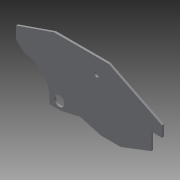
# Autodesk Inventor part: ShooterMountLeft_NERDS
Saved by Autodesk Inventor 2014 (Build 180170000, 170)
## iProperties
Created: 2016-01-30
Part Number: ShooterMountLeft_NERDS
Material: Generic
Document SubType Name: Modeling
Designer: bermudezr
Density: 1 g/cm^3
Appearance: Default
Author: bermudezr
Autodesk Inventor part; units mm, degrees
ref_plane "YZ Plane" through (0, 0, 0) normal (1, 0, 0) x (0, 1, 0)
ref_plane "XZ Plane" through (0, 0, 0) normal (0, 1, 0) x (-1, 0, 0)
ref_plane "XY Plane" through (0, 0, 0) normal (0, 0, 1) x (1, 0, 0)
sketch "Sketch1" plane through (0, 0, 0) normal (0, 0, 1) x (1, 0, 0)
  line L0 (-84.0821, 192.7052) -> (642.9929, 192.7052)
  line L1 (642.9929, 192.7052) -> (642.9929, -137.4948)
  line L2 (642.9929, -137.4948) -> (-84.0821, -137.4948)
  line L3 (-84.0821, -137.4948) -> (-84.0821, 192.7052)
  circle A0 centre (131.8179, -91.7748) radius 25.4
  circle A1 centre (318.0537, 116.5052) radius 12.7
  line L4 (642.9929, -137.4948) -> (592.1929, -137.4948)
  line L5 (592.1929, -137.4948) -> (592.1929, -73.9948)
  line L6 (592.1929, -73.9948) -> (642.9929, -73.9948)
  line L7 (642.9929, -73.9948) -> (642.9929, -137.4948)
  line L8 (642.9929, 192.7052) -> (592.6352, 192.7052)
  line L9 (642.9929, 2.2052) -> (642.9929, 192.7052)
  line L10 (-84.0821, 53.0052) -> (5.7204, 53.0052) construction
  line L11 (-84.0821, 65.7052) -> (68.3179, -137.4948)
  line L12 (595.3679, 192.7052) -> (595.3679, 2.2052)
  line L13 (595.3679, 2.2052) -> (642.9929, 2.2052)
  point P0 (0, 0)
  dimension "d0" = 727.075
  dimension "d2" = 50.8
  dimension "d3" = 25.4
  dimension "d4" = 215.9
  dimension "d5" = 279.4
  dimension "d14" = 152.4
  dimension "d15" = 203.2
  dimension "d16" = 330.2
  dimension "d17" = 63.5
  dimension "d19" = 50.8
  dimension "d20" = 139.7
  dimension "d21" = 45.72
  dimension "d22" = 254
  constraints: 28 end point, 5 parallel, 5 point on line, 4 horizontal, 3 perpendicular, 2 centre point
  measures "d0" distance of L1.end L2.end
  measures "d2" diameter of A0
  measures "d3" diameter of A1
  measures "d4" distance from line of L3 A0.centre
  measures "d5" distance of A1.centre A0.centre
  measures "d14" distance from line of L3 L11.end
  measures "d15" distance from line of L2 L11.start
  measures "d16" distance between parallel lines of L2 L0
  measures "d17" distance between parallel lines of L6 L2
  measures "d19" distance of L5.end L6.end
  measures "d20" distance between parallel lines of L13 L4
  measures "d21" distance from line of L2 A0.centre
  measures "d22" distance from line of L2 A1.centre
extrude "Extrusion1" add sketch "Sketch1" along normal blind 9.525 contours L0 L12 L13 L1 L6 L5 L2 L11 L3
sketch "Sketch3" plane through (0, 0, 9.525) normal (0, 0, 1) x (1, 0, 0)
  line L0 (595.3679, 2.2052) -> (595.3679, 192.7052) projected
  line L1 (595.3679, 192.7052) -> (-84.0821, 192.7052) projected
  line L2 (-84.0821, 192.7052) -> (-84.0821, 65.7052) projected
  line L3 (-84.0821, 127.1732) -> (106.4179, 192.7052)
  line L4 (595.3679, 2.2052) -> (684.2679, 2.2052)
  line L5 (684.2679, 2.2052) -> (684.2679, 40.3052)
  line L6 (684.2679, 40.3052) -> (595.3679, 40.3052)
  line L7 (595.3679, 40.3052) -> (595.3679, 2.2052)
  line L8 (684.2679, 40.3052) -> (379.4679, 192.7052)
  line L9 (595.3679, 40.3052) -> (595.3679, 84.7552)
  line L10 (595.3679, 84.7552) -> (595.3679, 192.7052)
  point P0 (0, 0)
  dimension "d32" = 190.5
  dimension "d33" = 65.532
  dimension "d38" = 88.9
  dimension "d39" = 38.1
  dimension "d40" = 215.9
  constraints: 16 end point, 5 point on line, 2 parallel, 1 collinear, 1 horizontal, 1 perpendicular
  measures "d32" distance from line of L2 L3.end
  measures "d33" distance from line of L1 L3.start
  measures "d38" distance of L6.end L5.end
  measures "d39" distance of L5.end L4.end
  measures "d40" distance of L0.end L8.end
extrude "Extrusion4" cut sketch "Sketch3" against normal blind 9.525 contours L3 L2 L1 | L8 L1 L0 | L0 L8 L6
sketch "Sketch4" plane through (0, 0, 9.525) normal (0, 0, 1) x (1, 0, 0)
  line L0 (595.3679, 2.2052) -> (595.3679, 84.7552) projected
  line L1 (595.3679, 84.7552) -> (379.4679, 192.7052) projected
  line L2 (595.3679, 84.7552) -> (684.2679, 40.3052)
  line L3 (684.2679, 40.3052) -> (595.3679, 40.3052)
  point P0 (0, 0)
  dimension "d43" = 88.9
  constraints: 4 end point, 1 collinear, 1 perpendicular, 1 point on line
  measures "d43" distance from line of L2.end L0
extrude "Extrusion5" add sketch "Sketch4" against normal blind 9.525
sketch "Sketch5" plane through (0, 0, 9.525) normal (0, 0, 1) x (1, 0, 0)
  line L0 (642.9929, 2.2052) -> (592.1929, 2.2052)
  line L1 (592.1929, 2.2052) -> (592.1929, -73.9948)
  line L2 (592.1929, -73.9948) -> (642.9929, -73.9948)
  line L3 (642.9929, -73.9948) -> (642.9929, 2.2052)
  point P0 (0, 0)
  constraints: 8 end point, 2 parallel, 1 horizontal, 1 perpendicular
extrude "Extrusion6" cut sketch "Sketch5" against normal blind 9.525
sketch "Sketch6" plane through (0, 0, 9.525) normal (0, 0, 1) x (1, 0, 0)
  line L0 (592.1929, -137.4948) -> (592.1929, 2.2052) projected
  line L1 (646.1679, 91.1052) -> (723.1394, 91.1052)
  line L2 (723.1394, 91.1052) -> (723.1394, -6.7385)
  line L3 (723.1394, -6.7385) -> (646.1679, -6.7385)
  line L4 (646.1679, -6.7385) -> (646.1679, 91.1052)
  line L5 (595.3679, 2.2052) -> (592.1929, 2.2052)
  line L6 (592.1929, 2.2052) -> (592.1929, 40.3052)
  line L7 (592.1929, 40.3052) -> (595.3679, 40.3052)
  line L8 (595.3679, 40.3052) -> (595.3679, 2.2052)
  point P0 (0, 0)
  dimension "d48" = 53.975
  constraints: 16 end point, 4 parallel, 2 horizontal, 2 perpendicular
  measures "d48" distance between parallel lines of L0 L4
extrude "Extrusion7" cut sketch "Sketch6" against normal blind 9.525
sketch "Sketch8" plane through (0, 0, 9.525) normal (0, 0, 1) x (1, 0, 0)
  line L0 (-84.0821, 65.7052) -> (68.3179, -137.4948) projected
  line L1 (68.3179, -137.4948) -> (592.1929, -137.4948) projected
  line L2 (592.1929, -137.4948) -> (592.1929, 40.3052) projected
  line L3 (592.1929, -96.6594) -> (439.7929, -137.4948)
  line L4 (341.7489, -137.4948) -> (170.3104, -117.1748)
  line L5 (170.3104, -117.1748) -> (53.0779, -117.1748)
  point P0 (0, 0)
  dimension "d51" = 152.4
  dimension "d52" = 165
  dimension "d53" = 98.044
  dimension "d54" = 20.32
  dimension "d60" = 173.24
  constraints: 6 end point, 4 point on line
  measures "d51" distance from line of L3.end L2
  measures "d52" angle of L1 L3
  measures "d53" distance of L3.end L4.start
  measures "d54" distance between parallel lines of L1 L5
  measures "d60" angle of L1 L4
extrude "Extrusion8" cut sketch "Sketch8" against normal blind 9.525
sketch "Sketch9" plane through (0, 0, 9.525) normal (0, 0, 1) x (1, 0, 0)
  line L0 (592.1929, -96.6594) -> (592.1929, 40.3052) projected
  line L1 (646.1679, 40.3052) -> (592.1929, 40.3052)
  line L2 (592.1929, 40.3052) -> (592.1929, 5.3802)
  line L3 (592.1929, 5.3802) -> (646.1679, 5.3802)
  line L4 (646.1679, 5.3802) -> (646.1679, 40.3052)
  point P0 (0, 0)
  dimension "d57" = 34.925
  constraints: 8 end point, 2 parallel, 1 horizontal, 1 perpendicular, 1 point on line
  measures "d57" distance of L2.end L1.end
extrude "Extrusion9" add sketch "Sketch9" against normal blind 9.525
sketch "Sketch10" plane through (0, 0, 9.525) normal (0, 0, 1) x (1, 0, 0)
  line L0 (-84.0821, 65.7052) -> (53.0779, -117.1748) projected
  line L1 (-84.0821, 127.1732) -> (-84.0821, 65.7052) projected
  line L2 (53.0779, -117.1748) -> (170.3104, -117.1748) projected
  arc A0 (82.3351, -98.9312) -> (-55.5071, 27.6052) centre (-44.6649, -98.9312) ccw
  line L3 (341.7489, -137.4948) -> (439.7929, -137.4948) projected
  line L4 (82.3351, -117.1748) -> (82.3351, -75.9981)
  point P0 (0, 0)
  point P1 (81.0179, -117.1748)
  point P2 (131.8179, -117.1748)
  dimension "d62" = 38.1
  dimension "d65" = 127
  dimension "d66" = 165.1
  constraints: 4 point on line, 2 end point, 2 point on circle, 1 centre point, 1 perpendicular, 1 tangent
  measures "d62" vertical distance of L0.start A0.end
  measures "d65" radius of A0
  measures "d66" distance from line of point (81.018, -117.175) L1
extrude "Extrusion10" cut sketch "Sketch10" against normal blind 25.4
sketch "Sketch12" plane through (0, 0, 9.525) normal (0, 0, 1) x (1, 0, 0)
  circle A0 centre (131.8179, -91.7748) radius 25.4 projected
  circle A1 centre (131.8179, -91.7748) radius 38.1
  point P0 (0, 0)
  dimension "d70" = 76.2
  constraints: 1 centre point, 1 coincident
  measures "d70" diameter of A1
extrude "Extrusion12" cut sketch "Sketch12" against normal blind 9.525
sketch "Sketch14" plane through (0, 0, 9.525) normal (0, 0, 1) x (1, 0, 0)
  arc A0 (160.2159, -117.1748) -> (103.4198, -117.1748) centre (131.8179, -91.7748) ccw projected
  line L0 (160.2159, -117.1748) -> (170.3104, -117.1748) projected
  line L1 (170.3104, -117.1748) -> (341.7489, -137.4948) projected
  line L2 (82.3351, -117.1748) -> (103.4198, -117.1748) projected
  circle A1 centre (131.8179, -91.7748) radius 38.1
  line L3 (341.7489, -137.4948) -> (82.3351, -137.4948)
  line L4 (82.3351, -137.4948) -> (82.3351, -117.1748)
  point P0 (0, 0)
  dimension "d74" = 20.32
  constraints: 4 end point, 1 coincident, 1 parallel, 1 perpendicular, 1 point on line, 3 other
  measures "d74" distance between parallel lines of L2 L3
extrude "Extrusion13" add sketch "Sketch14" against normal blind 9.525 contours L0 L1 L3 L4 L2 A1
sketch "Sketch15" plane through (0, 0, 9.525) normal (0, 0, 1) x (1, 0, 0)
  circle A0 centre (131.8179, -91.7748) radius 38.1 projected
  line L0 (82.3351, -98.9312) -> (82.3351, -137.4948) projected
  line L1 (82.3351, -137.4948) -> (439.7929, -137.4948) projected
  circle A1 centre (185.7929, -51.1348) radius 76.2
  circle A2 centre (373.8763, -101.9348) radius 76.2
  line L2 (82.3351, -110.8248) -> (177.5851, -110.8248)
  line L3 (177.5851, -110.8248) -> (177.5851, -72.7248)
  line L4 (177.5851, -72.7248) -> (82.3351, -72.7248)
  line L5 (82.3351, -72.7248) -> (82.3351, -110.8248)
  line L6 (236.6324, -107.8955) -> (341.4074, -137.4948)
  line L7 (-84.0821, 127.1732) -> (-84.0821, 65.7052) projected
  line L8 (131.8179, -129.8748) -> (175.334, -129.8748)
  line L9 (131.8179, -129.8748) -> (82.3351, -129.8748)
  line L10 (236.6324, -107.8955) -> (142.6601, -129.8748)
  point P0 (0, 0)
  point P1 (154.0824, -137.4948)
  dimension "d77" = 152.4
  dimension "d78" = 53.975
  dimension "d79" = 40.64
  dimension "d80" = 152.4
  dimension "d81" = 291.5412
  dimension "d82" = 35.56
  dimension "d84" = 95.25
  dimension "d85" = 38.1
  dimension "d86" = 26.67
  dimension "d87" = 82.55
  dimension "d90" = 104.775
  dimension "d101" = 60.325
  constraints: 16 end point, 5 point on line, 3 horizontal, 3 perpendicular, 2 parallel, 1 centre point, 1 vertical alignment, 4 other
  measures "d78" horizontal distance of point (185.793, -51.135) point (131.818, -91.775)
  measures "d79" vertical distance of point (131.818, -91.775) point (185.793, -51.135)
  measures "d80" diameter of A2
  measures "d81" distance from line of A2.centre L0
  measures "d82" distance from line of A2.centre L1
  measures "d84" distance of L4.end L3.end
  measures "d85" distance of L3.end L2.end
  measures "d86" distance between parallel lines of L2 L1
  measures "d87" horizontal distance of L6.start point (154.082, -137.495)
  measures "d90" horizontal distance of L6.end L6.start
  measures "d101" distance from line of L10.end L0
sketch "Sketch17" plane through (0, 0, 9.525) normal (0, 0, 1) x (1, 0, 0)
  line L0 (439.7929, -137.4948) -> (592.1929, -96.6594) projected
  line L1 (592.1929, -96.6594) -> (592.1929, 5.3802) projected
  line L2 (592.1929, -79.2096) -> (439.7929, -137.4948)
  point P0 (0, 0)
  dimension "d94" = 17.4498
  constraints: 2 end point, 1 point on line
  measures "d94" distance of L0.end L2.start
extrude "Extrusion16" cut sketch "Sketch17" against normal blind 9.525
extrude "Extrusion18" cut sketch "Sketch15" against normal blind 9.525 contours L8 L10 A1 L6 A2 L1 L0 L9 | L10 A1 | L6 L1 A2 picked at (315.3812, -131.2856)
sketch "Sketch20" plane through (0, 0, 9.525) normal (0, 0, 1) x (1, 0, 0)
  circle A0 centre (131.8179, -91.7748) radius 38.1 projected
  circle A1 centre (131.8179, -91.7748) radius 25.4
  point P0 (0, 0)
  dimension "d102" = 50.8
  constraints: 1 centre point, 1 coincident
  measures "d102" diameter of A1
extrude "Extrusion19" add sketch "Sketch20" against normal blind 9.525
sketch "Sketch21" plane through (0, 0, 9.525) normal (0, 0, 1) x (1, 0, 0)
  line L0 (-84.0821, 65.7052) -> (-55.5071, 27.6052) projected
  arc A0 (82.3351, -98.9312) -> (-55.5071, 27.6052) centre (-44.6649, -98.9312) ccw projected
  line L1 (-84.0821, 65.7052) -> (-43.4592, 28.0631)
  point P0 (0, 0)
  constraints: 2 end point, 1 point on circle
extrude "Extrusion20" cut sketch "Sketch21" against normal blind 9.525
body "Solid1"
